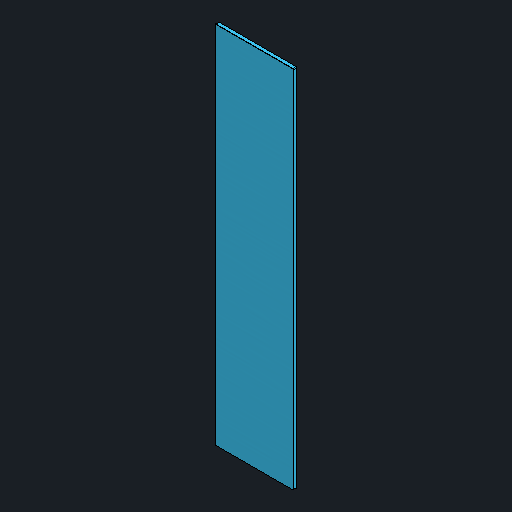
# Autodesk Inventor part: base-plate-for-bellows
Saved by Autodesk Inventor 2027.1 (Build 311270010, 270A)
## iProperties
Created: 2026-10-07
Part Number: base-plate-for-bellows
Material: Aluminum 6061
Document SubType Name: Modeling
Designer: queezz
Density: 2.7 g/cm^3
Appearance: Turquoise
Author: queezz
Autodesk Inventor part; units mm, degrees
ref_plane "YZ Plane" through (0, 0, 0) normal (1, 0, 0) x (0, 1, 0)
ref_plane "XZ Plane" through (0, 0, 0) normal (0, 1, 0) x (-1, 0, 0)
ref_plane "XY Plane" through (0, 0, 0) normal (0, 0, 1) x (1, 0, 0)
sketch "Sketch1" plane through (0, 0, 0) normal (0, 0, 1) x (1, 0, 0)
  line L0 (-107.5, 500) -> (107.5, 500)
  line L1 (107.5, 500) -> (107.5, -500)
  line L2 (107.5, -500) -> (-107.5, -500)
  line L3 (-107.5, -500) -> (-107.5, 500)
  point P0 (0, 0)
  point P1 (0, 500)
  point P2 (107.5, 0)
  dimension "d0" = 215
  dimension "d1" = 1000
  constraints: 8 end point, 2 midpoint, 2 parallel, 1 horizontal, 1 horizontal alignment, 1 perpendicular, 1 vertical alignment
  measures "d0" distance of L0.start L0.end
  measures "d1" distance of L0.end L1.end
extrude "Extrusion1" add sketch "Sketch1" along normal blind 10
fillet "Fillet1" radius 2 4 edges at (107.5, 500, 5) (-107.5, 500, 5) (107.5, -500, 5) (-107.5, -500, 5)
chamfer "Chamfer1" distance 0.5 angle 45 16 edges at (-107.5, 0, 10) (-106.9142, -499.4142, 10) (0, -500, 10) (106.9142, -499.4142, 10) (107.5, 0, 10) (106.9142, 499.4142, 10) (0, 500, 10) (-106.9142, 499.4142, 10) (-107.5, 0, 0) (-106.9142, -499.4142, 0) (0, -500, 0) (106.9142, -499.4142, 0) (107.5, 0, 0) (106.9142, 499.4142, 0) (0, 500, 0) (-106.9142, 499.4142, 0)
body "Solid1"
